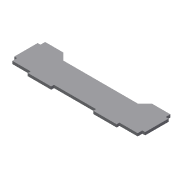
# Autodesk Inventor part: Lateral
Saved by Autodesk Inventor 2017 (Build 210142000, 142)
## iProperties
Created: 2017-06-24
Part Number: Lateral
Material: Generic
Document SubType Name: Modeling
Designer: Butri
Density: 1 g/cm^3
Appearance: Default
Author: Butri
Autodesk Inventor part; units mm, degrees
ref_plane "YZ Plane" through (0, 0, 0) normal (1, 0, 0) x (0, 1, 0)
ref_plane "XZ Plane" through (0, 0, 0) normal (0, 1, 0) x (-1, 0, 0)
ref_plane "XY Plane" through (0, 0, 0) normal (0, 0, 1) x (1, 0, 0)
sketch "Sketch1" plane through (0, 0, 0) normal (0, 0, 1) x (1, 0, 0)
  line L0 (280, 76) -> (280, 66) construction
  line L1 (280, 76) -> (274, 76) construction
  line L2 (274, 76) -> (274, 66) construction
  line L3 (280, 66) -> (274, 66) construction
  line L4 (280, 16) -> (280, 6) construction
  line L5 (280, 16) -> (274, 16) construction
  line L6 (274, 16) -> (274, 6) construction
  line L7 (280, 6) -> (274, 6) construction
  line L8 (235, 6) -> (235, 0) construction
  line L9 (235, 0) -> (280, 0) construction
  line L10 (280, 0) -> (280, 6) construction
  line L11 (235, 6) -> (280, 6) construction
  line L12 (95, 6) -> (95, 0) construction
  line L13 (95, 0) -> (185, 0) construction
  line L14 (185, 0) -> (185, 6) construction
  line L15 (95, 6) -> (185, 6) construction
  line L16 (45, 0) -> (45, 6) construction
  line L17 (0, 6) -> (45, 6) construction
  line L18 (0, 0) -> (0, 6) construction
  line L19 (0, 0) -> (45, 0) construction
  line L20 (0, 16) -> (0, 6) construction
  line L21 (0, 6) -> (6, 6) construction
  line L22 (6, 16) -> (6, 6) construction
  line L23 (0, 16) -> (6, 16) construction
  line L24 (0, 76) -> (0, 66) construction
  line L25 (0, 66) -> (6, 66) construction
  line L26 (6, 76) -> (6, 66) construction
  line L27 (0, 76) -> (6, 76) construction
  line L28 (274, 16) -> (280, 16)
  line L29 (280, 16) -> (280, 66)
  line L30 (280, 66) -> (274, 66)
  line L31 (6, 16) -> (0, 16)
  line L32 (0, 16) -> (0, 66)
  line L33 (0, 66) -> (6, 66)
  line L34 (95, 6) -> (95, 0)
  line L35 (95, 0) -> (45, 0)
  line L36 (45, 0) -> (45, 6)
  line L37 (185, 6) -> (185, 0)
  line L38 (185, 0) -> (235, 0)
  line L39 (235, 0) -> (235, 6)
  line L40 (274, 76) -> (274, 66)
  line L41 (274, 16) -> (274, 6)
  line L42 (274, 6) -> (235, 6)
  line L43 (185, 6) -> (95, 6)
  line L44 (45, 6) -> (6, 6)
  line L45 (6, 6) -> (6, 16)
  line L46 (6, 66) -> (6, 76)
  line L47 (45, 76) -> (45, 61)
  line L48 (45, 61) -> (235, 61)
  line L49 (235, 61) -> (235, 76)
  line L50 (6, 76) -> (45, 76)
  line L51 (235, 76) -> (274, 76)
extrude "Extrusion1" add sketch "Sketch1" against normal blind 6
chamfer "Chamfer1" distance 15 angle 45 2 edges at (45, 61, -3) (235, 61, -3)
body "Solid1"
